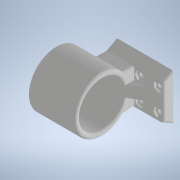
# Autodesk Inventor part: mot137
Saved by Autodesk Inventor 2022 (Build 260153000, 153)
## iProperties
Part Number: mot137
Material: Типовые
Document SubType Name: Modeling
Designer: korsh
Density: 1 g/cm^3
Appearance: По умолчанию
Author: korsh
Autodesk Inventor part; units mm, degrees
ref_plane "YZ Plane" through (0, 0, 0) normal (1, 0, 0) x (0, 1, 0)
ref_plane "XZ Plane" through (0, 0, 0) normal (0, 1, 0) x (-1, 0, 0)
ref_plane "XY Plane" through (0, 0, 0) normal (0, 0, 1) x (1, 0, 0)
sketch "Эскиз2" plane through (36.9468, 10.3967, 35.0196) normal (-1, 0, 0) x (0, -1, 0)
  circle A0 centre (-8.1033, -16.5196) radius 12.5 projected
  circle A1 centre (-8.1033, -16.5196) radius 18.4 projected
  circle A2 centre (-21.5267, -24.2696) radius 1.5 projected
  circle A3 centre (-8.1032, -32.0196) radius 1.5 projected
  circle A4 centre (5.3201, -24.2696) radius 1.5 projected
  circle A5 centre (5.3201, -8.7696) radius 1.5 projected
  circle A6 centre (-8.1033, -1.0196) radius 1.5 projected
  circle A7 centre (-21.5266, -8.7696) radius 1.5 projected
  circle A8 centre (-1.1033, -16.5196) radius 8 projected
  circle A9 centre (-1.1032, -16.5197) radius 6.0001 projected
  circle A10 centre (-1.1032, -16.5197) radius 4.5001 projected
  point P0 (10.3967, -35.0196)
extrude "Выдавливание1" add sketch "Эскиз2" along normal blind 3 contours A1
sketch "Эскиз3" plane through (33.9468, 18.5, 18.5) normal (-1, 0, 0) x (0, 0, 1)
  circle A0 centre (0, 0) radius 18.4 projected
  circle A1 centre (0, 0) radius 21.5
  point P0 (-18.5, -18.5)
  dimension "d2" = 43
  constraints: 1 centre point, 1 coincident
  measures "d2" diameter of A1
extrude "Выдавливание2" add sketch "Эскиз3" against normal blind 25
sketch "Эскиз5" plane through (33.9468, 18.5, 18.5) normal (-1, 0, 0) x (0, 0, 1)
  line L0 (-1.5, 12) -> (1.5, 12) projected
  arc A0 (7.3795, -10.0892) -> (-7.3794, -10.0893) centre (0, 0) ccw projected
  line L1 (0, 36.5204) -> (-20, 36.5204)
  line L2 (-20, 36.5204) -> (0, 0)
  line L3 (0, 36.5204) -> (20, 36.5204)
  line L4 (20, 36.5204) -> (0, 0)
  circle A1 centre (0, 0) radius 21.5 projected
  arc A2 (10.3271, 18.8574) -> (-10.327, 18.8574) centre (0, 0) ccw
  point P0 (-18.5, -18.5)
  dimension "d7" = 20
  dimension "d8" = 20
  constraints: 8 end point, 4 point on circle, 2 horizontal, 2 point on line, 1 centre point, 1 equal radius
  measures "d7" distance of L1.start L1.end
  measures "d8" distance of L1.start L3.end
extrude "Выдавливание3" add sketch "Эскиз5" against normal blind 50 contours A1 L2 L1 L3 L4
sketch "Эскиз6" plane through (33.9468, 10.3967, 35.0196) normal (-1, 0, 0) x (0, 0, 1)
  line L0 (3.4804, 44.6237) -> (-36.5196, 44.6237) projected
  arc A0 (-26.8467, 26.9607) -> (-6.1926, 26.9607) centre (-16.5196, 8.1033) ccw projected
  line L1 (-6.1926, 26.9607) -> (3.4804, 44.6237) projected
  line L2 (3.4804, 44.6237) -> (-36.5196, 44.6237) projected
  line L3 (-36.5196, 44.6237) -> (-26.8467, 26.9607) projected
  circle A1 centre (-8.7696, -5.3201) radius 1.5 projected
  circle A2 centre (-1.0196, 8.1033) radius 1.5 projected
  circle A3 centre (-24.2696, -5.3201) radius 1.5 projected
  circle A4 centre (-32.0196, 8.1032) radius 1.5 projected
  circle A5 centre (-8.7696, 21.5266) radius 1.5 projected
  circle A6 centre (-24.2696, 21.5267) radius 1.5 projected
  arc A7 (-9.1401, -1.9859) -> (-23.899, -1.9861) centre (-16.5196, 8.1033) ccw projected
  arc A8 (-23.899, -1.9861) -> (-9.1401, -1.9859) centre (-16.5196, 1.1033) ccw projected
  line L4 (-33.5196, 43.3095) -> (0.4804, 43.3095)
  line L5 (-33.5196, 43.3095) -> (-25.7696, 29.0831)
  line L6 (0.4804, 43.3095) -> (-7.3011, 29.1003)
  line L7 (-6.1926, 26.9607) -> (3.4804, 44.6237) projected
  arc A9 (-7.3011, 29.1003) -> (-25.7696, 29.0831) centre (-16.5215, 14.2207) ccw
  point P0 (-35.0196, -10.3967)
  dimension "d11" = 34
  dimension "d12" = 2
  dimension "d13" = 2
  constraints: 6 end point, 2 point on circle, 1 centre point, 1 horizontal, 1 parallel
  measures "d11" distance of L4.start L4.end
  measures "d12" distance from line of L1 L4.end
  measures "d13" distance from line of L3 L4.start
extrude "Выдавливание4" cut sketch "Эскиз6" against normal blind 1 contours L4 L6 A9 L5
sketch "Эскиз8" plane through (83.9468, 18.5, 18.5) normal (1, 0, 0) x (0, 0, -1)
  arc A0 (-10.3271, 18.8574) -> (10.327, 18.8574) centre (0, 0) ccw projected
  arc A1 (10.327, 18.8574) -> (-10.3271, 18.8574) centre (0, 0) ccw projected
  arc A2 (10.327, 18.8574) -> (-10.3271, 18.8574) centre (0, 0) ccw
  line L0 (10.327, 18.8574) -> (20, 36.5204) projected
  line L1 (15.1635, 27.6889) -> (-15.1635, 27.6889)
  line L2 (-10.3271, 18.8574) -> (-20, 36.5204) projected
  line L3 (-15.1635, 27.6889) -> (-10.3271, 18.8574)
  line L4 (15.1635, 27.6889) -> (10.327, 18.8574)
  point P0 (18.5, -18.5)
  constraints: 6 end point, 2 collinear, 2 midpoint, 2 point on circle, 1 centre point
extrude "Выдавливание5" cut sketch "Эскиз8" against normal blind 25 contours L2 L1 L0 A1
sketch "Эскиз9" plane through (83.9468, 46.1889, 3.3365) normal (0, -1, -0.0000002) x (1, 0, 0)
  line L0 (0, 30.327) -> (0, 0) projected
  line L1 (-25, 30.327) -> (0, 30.327) projected
  line L2 (-25, 30.327) -> (-25, 0) projected
  line L3 (0, 0) -> (-25, 0) projected
  line L4 (0, 0) -> (-25, 30.327) construction
  line L5 (-25, 30.327) -> (0, 30.327) projected
  line L6 (-25, 30.327) -> (-25, 0) projected
  line L7 (0, 30.327) -> (-25, 0) construction
  circle A0 centre (-4.5, 5.4589) radius 2
  circle A1 centre (-20.5, 5.4589) radius 2
  circle A2 centre (-20.5, 24.8682) radius 2
  circle A3 centre (-4.5, 24.8682) radius 2
  point P0 (-83.9468, -3.3365)
  dimension "d19" = 4
  dimension "d20" = 4
  dimension "d21" = 4
  dimension "d22" = 4
  dimension "d23" = 4.5
  dimension "d24" = 4.5
  dimension "d25" = 4.5
  dimension "d26" = 4.5
  constraints: 4 centre point, 4 end point, 4 point on line
  measures "d19" diameter of A0
  measures "d20" diameter of A1
  measures "d21" diameter of A2
  measures "d22" diameter of A3
  measures "d23" distance from line of L0 A0.centre
  measures "d24" distance from line of L0 A3.centre
  measures "d25" distance from line of L2 A1.centre
  measures "d26" distance from line of L2 A2.centre
extrude "Выдавливание6" cut sketch "Эскиз9" against normal blind 25 contours A0 | A1 | A2 | A3
sketch "Эскиз11" plane through (83.9468, 46.1889, 3.3365) normal (0, -1, -0.0000002) x (1, 0, 0)
  circle A0 centre (-20.5, 5.4589) radius 2 projected
  circle A1 centre (-20.5, 24.8682) radius 2 projected
  circle A2 centre (-4.5, 24.8682) radius 2 projected
  circle A3 centre (-4.5, 5.4589) radius 2 projected
  line L0 (-17.1203, 7.8791) -> (-16.7142, 3.742)
  line L1 (-16.7142, 3.742) -> (-20.0939, 1.3218)
  line L2 (-20.0939, 1.3218) -> (-23.8797, 3.0387)
  line L3 (-23.8797, 3.0387) -> (-24.2858, 7.1757)
  line L4 (-24.2858, 7.1757) -> (-20.9061, 9.5959)
  line L5 (-20.9061, 9.5959) -> (-17.1203, 7.8791)
  line L6 (-18.4339, 21.2611) -> (-22.5908, 21.2753)
  line L7 (-22.5908, 21.2753) -> (-24.6569, 24.8824)
  line L8 (-24.6569, 24.8824) -> (-22.5661, 28.4753)
  line L9 (-22.5661, 28.4753) -> (-18.4092, 28.461)
  line L10 (-18.4092, 28.461) -> (-16.3431, 24.8539)
  line L11 (-16.3431, 24.8539) -> (-18.4339, 21.2611)
  line L12 (-7.9629, 22.5686) -> (-8.223, 26.7174)
  line L13 (-8.223, 26.7174) -> (-4.76, 29.017)
  line L14 (-4.76, 29.017) -> (-1.0371, 27.1677)
  line L15 (-1.0371, 27.1677) -> (-0.777, 23.019)
  line L16 (-0.777, 23.019) -> (-4.24, 20.7194)
  line L17 (-4.24, 20.7194) -> (-7.9629, 22.5686)
  line L18 (-7.0942, 8.707) -> (-2.9842, 9.3296)
  line L19 (-2.9842, 9.3296) -> (-0.39, 6.0815)
  line L20 (-0.39, 6.0815) -> (-1.9058, 2.2108)
  line L21 (-1.9058, 2.2108) -> (-6.0158, 1.5882)
  line L22 (-6.0158, 1.5882) -> (-8.61, 4.8363)
  line L23 (-8.61, 4.8363) -> (-7.0942, 8.707)
  point P0 (-83.9468, -3.3365)
  dimension "d29" = 7.2
  dimension "d30" = 7.2
  dimension "d31" = 7.2
  dimension "d32" = 7.2
  constraints: 48 end point, 4 coincident, 3 point on line, 52 other
  measures "d29" distance between parallel lines of L2 L5
  measures "d30" distance between parallel lines of L11 L8
  measures "d31" distance between parallel lines of L12 L15
  measures "d32" distance between parallel lines of L22 L19
extrude "Выдавливание7" cut sketch "Эскиз11" against normal blind 2
sketch "Эскиз12" plane through (58.9468, 18.5, 18.5) normal (1, 0, 0) x (0, 0, -1)
  circle A0 centre (0, 0) radius 18.4 projected
  arc A1 (-10.3271, 18.8574) -> (10.327, 18.8574) centre (0, 0) ccw projected
  line L0 (15.1635, 27.6889) -> (10.327, 18.8574) projected
  line L1 (-15.1635, 27.6889) -> (15.1635, 27.6889) projected
  line L2 (-10.3271, 18.8574) -> (-15.1635, 27.6889) projected
  line L3 (-15.1635, 27.6889) -> (15.1635, 27.6889) projected
  line L4 (-15.1635, 27.6889) -> (-15.5767, 14.8195)
  arc A2 (-10.3271, 18.8574) -> (10.327, 18.8574) centre (0, 0) ccw projected
  line L5 (-10.3271, 18.8574) -> (-15.1635, 27.6889) projected
  line L6 (-15.1635, 27.6889) -> (-10.3271, 18.8574)
  arc A3 (-10.3271, 18.8574) -> (-15.5767, 14.8195) centre (0, 0) ccw
  line L7 (15.1635, 27.6889) -> (16.2208, 14.1115)
  line L8 (20, 36.5204) -> (10.327, 18.8574) projected
  line L9 (15.1635, 27.6889) -> (10.327, 18.8574)
  arc A4 (16.2208, 14.1115) -> (10.327, 18.8574) centre (0, 0) ccw
  point P0 (18.5, -18.5)
  constraints: 8 end point, 8 point on circle, 2 centre point, 2 collinear, 2 concentric
extrude "Выдавливание8" add sketch "Эскиз12" against normal blind 15 contours A1 L4 L2 | A1 L0 L7
sketch "Эскиз13" plane through (83.9468, 46.1889, 3.3365) normal (0, -1, -0.0000002) x (1, 0, 0)
  line L0 (-25, 30.327) -> (-25, 0) projected
  line L1 (-25, 16.6635) -> (-10, 16.6635)
  line L2 (-10, 16.6635) -> (-10, 13.6635)
  line L3 (-10, 13.6635) -> (-25, 13.6635)
  line L4 (-25, 13.6635) -> (-25, 16.6635)
  line L5 (-25, 30.327) -> (0, 30.327) projected
  line L6 (0, 0) -> (-25, 0) projected
  point P0 (-83.9468, -3.3365)
  dimension "d37" = 15
  dimension "d38" = 3
  dimension "d39" = 13.6635
  dimension "d40" = 30.327
  constraints: 8 end point, 2 parallel, 1 horizontal, 1 perpendicular, 1 point on line
  measures "d37" distance of L2.end L3.end
  measures "d38" distance of L1.end L2.end
  measures "d39" distance between parallel lines of L1 L5
  measures "d40" distance between parallel lines of L6 L5
extrude "Выдавливание9" add sketch "Эскиз13" along normal blind 8.5
sketch "Эскиз14" plane through (73.9468, 46.1889, 17) normal (0, 0.0000002, -1) x (-1, 0, 0)
  line L0 (15, -8.5) -> (0, -8.5) projected
  line L1 (0, 0) -> (0, -8.5) projected
  line L2 (15, -8.5) -> (0, 0)
  line L3 (0, 0) -> (0, -8.5)
  line L4 (0, -8.5) -> (15, -8.5)
  point P0 (73.9468, -46.1889)
  constraints: 6 end point, 1 collinear, 1 perpendicular
extrude "Выдавливание10" cut sketch "Эскиз14" against normal blind 8.5
sketch "Эскиз16" plane through (33.9468, 55.0204, 38.5) normal (0, 1, 0) x (1, 0, 0)
  point P0 (-33.9468, 38.5)
sketch "Эскиз17" plane through (58.9468, 18.5, 18.5) normal (1, 0, 0) x (0, 0, -1)
  circle A0 centre (0, 0) radius 18.4 projected
  circle A1 centre (0, 0) radius 19.4
  point P0 (18.5, -18.5)
  dimension "d45" = 38.8
  constraints: 1 centre point, 1 coincident
  measures "d45" diameter of A1
extrude "Выдавливание11" cut sketch "Эскиз17" against normal blind 22
sketch "Эскиз18" plane through (58.9468, 18.5, 18.5) normal (1, 0, 0) x (0, 0, -1)
  arc A0 (-1.5, 19.3419) -> (1.5, 19.3419) centre (0, 0) ccw projected
  line L0 (-1.5, 19.3419) -> (-1.5, 27.6889) projected
  line L1 (-15.1635, 27.6889) -> (-1.5, 27.6889) projected
  line L2 (-15.1635, 27.6889) -> (-15.5767, 14.8195) projected
  arc A1 (-15.5767, 14.8195) -> (16.2208, 14.1115) centre (0, 0) ccw projected
  line L3 (16.2208, 14.1115) -> (15.1635, 27.6889) projected
  line L4 (1.5, 27.6889) -> (15.1635, 27.6889) projected
  line L5 (1.5, 27.6889) -> (1.5, 19.3419) projected
  line L6 (16.2208, 14.1115) -> (15.1635, 27.6889) projected
  line L7 (15.9334, 17.8018) -> (16.2208, 14.1115)
  line L8 (-15.5767, 14.8195) -> (-15.4679, 18.2078)
  line L9 (-15.5767, 14.8195) -> (-15.1635, 27.6889) projected
  arc A2 (1.5, 23.8439) -> (-1.5, 23.8438) centre (0, 0) ccw
  arc A3 (-15.4679, 18.2078) -> (15.9334, 17.8018) centre (0, 0) ccw
  point P0 (18.5, -18.5)
  constraints: 4 end point, 4 point on circle, 4 point on line, 2 centre point, 1 coincident, 1 collinear
extrude "Выдавливание12" add sketch "Эскиз18" against normal blind 25 contours L2 A1 L3 A3
sketch "Эскиз19" plane through (43.9468, 18.5, 18.5) normal (-1, 0, 0) x (0, 0, 1)
  arc A0 (-10.327, 18.8574) -> (-16.2208, 14.1115) centre (0, 0) ccw projected
  line L0 (-15.1635, 27.6889) -> (-10.327, 18.8574) projected
  line L1 (-15.1635, 27.6889) -> (-15.9334, 17.8018) projected
  line L2 (-15.9334, 17.8018) -> (-16.2208, 14.1115) projected
  line L3 (10.3271, 18.8574) -> (15.1635, 27.6889) projected
  arc A1 (15.5767, 14.8195) -> (10.3271, 18.8574) centre (0, 0) ccw projected
  line L4 (15.5767, 14.8195) -> (15.4679, 18.2078) projected
  line L5 (15.4679, 18.2078) -> (15.1635, 27.6889) projected
  point P0 (-18.5, -18.5)
extrude "Выдавливание13" add sketch "Эскиз19" along normal blind 10
sketch "Эскиз20" plane through (73.9468, 46.1889, 17) normal (0, 0.0000002, -1) x (-1, 0, 0)
  line L0 (0, 0) -> (15, -8.5) projected
  line L1 (15, -8.347) -> (15, -8.5) projected
  line L2 (15, 0) -> (15, -8.347) projected
  line L3 (0, 0) -> (15, 0) projected
  point P0 (73.9468, -46.1889)
extrude "Выдавливание14" add sketch "Эскиз20" along normal blind 3.5
sketch "Эскиз21" plane through (58.9468, 46.1889, 20) normal (0, -0.0000002, 1) x (1, 0, 0)
  line L0 (0, -8.5) -> (15, 0) projected
  line L1 (0, 0) -> (15, 0) projected
  line L2 (0, -8.347) -> (0, 0) projected
  line L3 (0, -8.5) -> (0, -8.347) projected
  point P0 (-58.9468, -46.1889)
extrude "Выдавливание15" add sketch "Эскиз21" along normal blind 3.5
sketch "Эскиз22" plane through (34.9468, 10.3967, 35.0196) normal (-1, 0, 0) x (0, 0, 1)
  line L0 (-33.5196, 43.3095) -> (0.4804, 43.3095) projected
  line L1 (-25.7696, 29.0831) -> (-33.5196, 43.3095) projected
  arc A0 (-7.3011, 29.1003) -> (-25.7696, 29.0831) centre (-16.5215, 14.2207) ccw projected
  line L2 (0.4804, 43.3095) -> (-7.3011, 29.1003) projected
  point P0 (-35.0196, -10.3967)
  point P1 (-10.9637, 37.7922)
extrude "Выдавливание16" add sketch "Эскиз22" along normal blind 1
fillet "Сопряжение1" radius 2 2 edges at (58.9468, 31.1687, 3.8077) (58.9468, 3.8077, 31.1687)
fillet "Сопряжение2" radius 2 12 edges at (66.0548, 41.7168, 13.5) (66.0548, 41.7168, 23.5) (58.9468, 41.2454, 2.9515) (58.9468, -5.389, 18.8088) (58.9468, 41.4484, 33.8157) (83.9468, 50.6047, 0.9182) (83.9468, 46.1889, 18.5) (83.9468, 50.6047, 36.0818) (33.9468, 50.6047, 36.0818) (33.9468, 41.4484, 33.8157) (33.9468, 41.2454, 2.9515) (33.9468, 50.6047, 0.9182)
sketch "Эскиз31" plane through (33.9468, 10.3967, 35.0196) normal (-1, 0, 0) x (0, 0, 1)
  arc A0 (-30.3143, 27.6093) -> (-3.1028, 27.8711) centre (-16.5196, 8.1033) ccw projected
  line L0 (-3.3726, 36.2739) -> (-3.1028, 27.8711) projected
  line L1 (1.2001, 44.6237) -> (-3.3726, 36.2739) projected
  line L2 (1.2001, 44.6237) -> (-34.2393, 44.6237) projected
  line L3 (-29.6429, 36.2306) -> (-34.2393, 44.6237) projected
  line L4 (-30.3143, 27.6093) -> (-29.6429, 36.2306) projected
  circle A1 centre (-8.7696, -5.3201) radius 1.5 projected
  circle A2 centre (-1.0196, 8.1033) radius 1.5 projected
  circle A3 centre (-24.2696, -5.3201) radius 1.5 projected
  circle A4 centre (-32.0196, 8.1032) radius 1.5 projected
  circle A5 centre (-8.7696, 21.5266) radius 1.5 projected
  circle A6 centre (-24.2696, 21.5267) radius 1.5 projected
  arc A7 (-9.1401, -1.9859) -> (-23.899, -1.9861) centre (-16.5196, 8.1033) ccw projected
  arc A8 (-23.899, -1.9861) -> (-9.1401, -1.9859) centre (-16.5196, 1.1033) ccw projected
  circle A9 centre (-16.5196, 8.1033) radius 23.891
  point P0 (-35.0196, -10.3967)
  constraints: 1 coincident, 3 other
extrude "Выдавливание26" add sketch "Эскиз31" along normal blind 15 contours A9 A0
sketch "Эскиз32" plane through (36.9468, 18.5, 18.5) normal (1, 0, 0) x (0, 0, -1)
  circle A0 centre (0, 0) radius 19.4 projected
  arc A1 (7.3794, -10.0893) -> (-7.3795, -10.0892) centre (0, 0) ccw projected
  arc A2 (-7.3795, -10.0892) -> (7.3794, -10.0893) centre (-0.0001, -7) ccw projected
  circle A3 centre (7.7499, 13.4234) radius 1.5 projected
  circle A4 centre (-7.75, 13.4234) radius 1.5 projected
  circle A5 centre (15.5, 0) radius 1.5 projected
  circle A6 centre (7.75, -13.4234) radius 1.5 projected
  circle A7 centre (-15.5, 0) radius 1.5 projected
  circle A8 centre (-7.7501, -13.4234) radius 1.5 projected
  point P0 (18.5, -18.5)
extrude "Выдавливание27" cut sketch "Эскиз32" against normal blind 15
